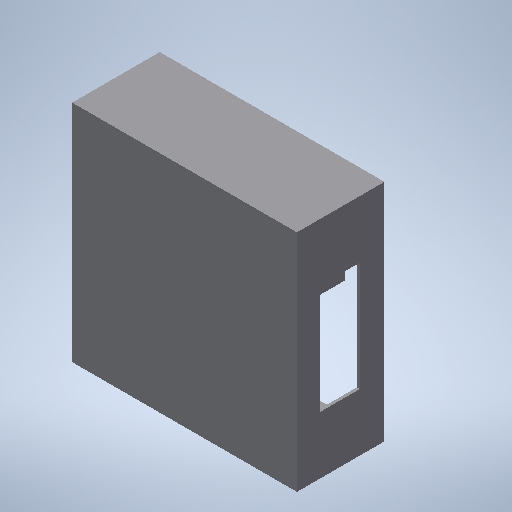
# Autodesk Inventor part: 零件1
Saved by Autodesk Inventor 2025 (Build 290162000, 162)
## iProperties
Created: 2024-03-26
Part Number: 零件1
Material: 常规
Document SubType Name: Modeling
Designer: Administrator
Density: 1 g/cm^3
Appearance: 默认
Author: Administrator
Autodesk Inventor part; units mm, degrees
ref_plane "YZ Plane" through (0, 0, 0) normal (1, 0, 0) x (0, 1, 0)
ref_plane "XZ Plane" through (0, 0, 0) normal (0, 1, 0) x (-1, 0, 0)
ref_plane "XY Plane" through (0, 0, 0) normal (0, 0, 1) x (1, 0, 0)
sketch "草图1" plane through (0, 0, 0) normal (0, 1, 0) x (-1, 0, 0)
  line L0 (75, 0) -> (75, -75)
  line L1 (75, -75) -> (-75, -75)
  line L2 (-75, -75) -> (-75, 75)
  line L3 (-75, 75) -> (75, 75)
  line L4 (75, 75) -> (75, 0)
  line L5 (77, 0) -> (77, 77)
  line L6 (77, 77) -> (-77, 77)
  line L7 (-77, 77) -> (-77, -77)
  line L8 (-77, -77) -> (77, -77)
  line L9 (77, -77) -> (77, 0)
  line L10 (75, 0) -> (75, 27)
  line L11 (75, 27) -> (7, 27)
  line L12 (7, 27) -> (7, -27)
  line L13 (7, -27) -> (75, -27)
  line L14 (75, -27) -> (75, -29)
  line L15 (75, -29) -> (5, -29)
  line L16 (5, -29) -> (5, 29)
  line L17 (5, 29) -> (75, 29)
  point P0 (0, 0)
  dimension "d2" = 150
  dimension "d3" = 150
  dimension "d4" = 150
  dimension "d6" = 77
  dimension "d7" = 154
  dimension "d8" = 154
  dimension "d9" = 154
  dimension "d14" = 70
  constraints: 36 end point, 6 perpendicular, 4 parallel, 4 point on line
  measures "d2" distance of L0.end L1.end
  measures "d3" distance of L1.end L2.end
  measures "d4" distance of L2.end L3.end
  measures "d6" distance of L5.start L5.end
  measures "d7" distance of L5.end L6.end
  measures "d8" distance of L6.end L7.end
  measures "d9" distance of L7.end L8.end
  measures "d14" distance of L14.end L15.end
sketch "草图2" plane through (0, 0, 0) normal (0, 1, 0) x (-1, 0, 0)
  line L0 (75, 0) -> (75, -75)
  line L1 (75, -75) -> (-75, -75)
  line L2 (-75, -75) -> (-75, 75)
  line L3 (-75, 75) -> (75, 75)
  line L4 (75, 75) -> (75, 0)
  line L5 (77, 0) -> (77, 77)
  line L6 (77, 77) -> (-77, 77)
  line L7 (-77, 77) -> (-77, -77)
  line L8 (-77, -77) -> (77, -77)
  line L9 (77, -77) -> (77, 0)
  line L10 (75, 0) -> (75, 27)
  line L11 (75, 27) -> (7, 27)
  line L12 (7, 27) -> (7, -27)
  line L13 (7, -27) -> (75, -27)
  line L14 (75, -27) -> (75, -29)
  line L15 (75, -29) -> (5, -29)
  line L16 (5, -29) -> (5, 29)
  line L17 (5, 29) -> (75, 29)
  line L18 (75, 0) -> (75, -75)
  line L19 (75, -75) -> (-75, -75)
  line L20 (-75, -75) -> (-75, 75)
  line L21 (-75, 75) -> (75, 75)
  line L22 (75, 75) -> (75, 0)
  line L23 (77, 0) -> (77, 77)
  line L24 (77, 77) -> (-77, 77)
  line L25 (-77, 77) -> (-77, -77)
  line L26 (-77, -77) -> (77, -77)
  line L27 (77, -77) -> (77, 0)
  line L28 (75, 0) -> (75, 27)
  line L29 (75, 27) -> (7, 27)
  line L30 (7, 27) -> (7, -27)
  line L31 (7, -27) -> (75, -27)
  line L32 (75, -27) -> (75, -29)
  line L33 (75, -29) -> (5, -29)
  line L34 (5, -29) -> (5, 29)
  line L35 (5, 29) -> (75, 29)
  point P0 (0, 0)
  point P1 (0, 0)
  point P2 (0, 0)
  dimension "d16" = 150
  dimension "d17" = 150
  dimension "d18" = 150
  dimension "d19" = 77
  dimension "d20" = 154
  dimension "d21" = 154
  dimension "d22" = 154
  dimension "d23" = 70
  dimension "d24" = 150
  dimension "d25" = 150
  dimension "d26" = 150
  dimension "d27" = 77
  dimension "d28" = 154
  dimension "d29" = 154
  dimension "d30" = 154
  dimension "d31" = 70
  constraints: 72 end point, 12 perpendicular, 8 parallel, 8 point on line
  measures "d16" distance of L0.end L1.end
  measures "d17" distance of L1.end L2.end
  measures "d18" distance of L2.end L3.end
  measures "d19" distance of L5.start L5.end
  measures "d20" distance of L5.end L6.end
  measures "d21" distance of L6.end L7.end
  measures "d22" distance of L7.end L8.end
  measures "d23" distance of L14.end L15.end
  measures "d24" distance of L18.end L19.end
  measures "d25" distance of L19.end L20.end
  measures "d26" distance of L20.end L21.end
  measures "d27" distance of L23.start L23.end
  measures "d28" distance of L23.end L24.end
  measures "d29" distance of L24.end L25.end
  measures "d30" distance of L25.end L26.end
  measures "d31" distance of L32.end L33.end
sketch "草图3" plane through (0, 0, 0) normal (0, 1, 0) x (-1, 0, 0)
  line L0 (75, 0) -> (75, -75)
  line L1 (75, -75) -> (-75, -75)
  line L2 (-75, -75) -> (-75, 75)
  line L3 (-75, 75) -> (75, 75)
  line L4 (75, 75) -> (75, 0)
  line L5 (77, 0) -> (77, 77)
  line L6 (77, 77) -> (-77, 77)
  line L7 (-77, 77) -> (-77, -77)
  line L8 (-77, -77) -> (77, -77)
  line L9 (77, -77) -> (77, 0)
  line L10 (75, 0) -> (75, 27)
  line L11 (75, 27) -> (7, 27)
  line L12 (7, 27) -> (7, -27)
  line L13 (7, -27) -> (75, -27)
  line L14 (75, -27) -> (75, -29)
  line L15 (75, -29) -> (5, -29)
  line L16 (5, -29) -> (5, 29)
  line L17 (5, 29) -> (75, 29)
  point P0 (0, 0)
  point P1 (0, 0)
  dimension "d32" = 150
  dimension "d33" = 150
  dimension "d34" = 150
  dimension "d35" = 77
  dimension "d36" = 154
  dimension "d37" = 154
  dimension "d38" = 154
  dimension "d39" = 70
  constraints: 36 end point, 6 perpendicular, 4 parallel, 4 point on line
  measures "d32" distance of L0.end L1.end
  measures "d33" distance of L1.end L2.end
  measures "d34" distance of L2.end L3.end
  measures "d35" distance of L5.start L5.end
  measures "d36" distance of L5.end L6.end
  measures "d37" distance of L6.end L7.end
  measures "d38" distance of L7.end L8.end
  measures "d39" distance of L14.end L15.end
extrude "拉伸3" add sketch "草图3" along normal blind 5 contours L0 L15 L16 L17 L4 L11 L12 L13 | L9 L8 L7 L6 L5
extrude "拉伸4" add sketch "草图2" along normal blind 50
extrude "拉伸5" add sketch "草图1" against normal blind 10 contours L0 L13 L12 L11 L4 | L0 L15 L16 L17 L4 L11 L12 L13 | L0 L1 L2 L3 L4 L17 L16 L15 | L9 L8 L7 L6 L5
sketch "草图4" plane through (77, 50, 77) normal (1, 0, 0) x (0, 0, -1)
  line L0 (77, -44) -> (114.5, -44)
  line L1 (114.5, -44) -> (114.5, -17)
  line L2 (114.5, -17) -> (39.5, -17)
  line L3 (39.5, -17) -> (39.5, -44)
  line L4 (39.5, -44) -> (77, -44)
  point P0 (77, -50)
  dimension "d53" = 27
  dimension "d54" = 75
  constraints: 10 end point
  measures "d53" distance of L0.end L1.end
  measures "d54" distance of L1.end L2.end
extrude "拉伸6" cut sketch "草图4" against normal blind 3
sketch "草图5" plane through (-77, 50, -77) normal (-1, 0, 0) x (0, 0, 1)
  line L0 (154, -60) -> (0, -60) projected
  line L1 (77, -50) -> (104, -50)
  line L2 (104, -50) -> (104, -40)
  line L3 (104, -40) -> (50, -40)
  line L4 (50, -40) -> (50, -50)
  line L5 (50, -50) -> (77, -50)
  dimension "d58" = 10
  dimension "d59" = 54
  constraints: 10 end point, 2 parallel, 2 perpendicular, 1 collinear
  measures "d58" distance of L1.end L2.end
  measures "d59" distance of L2.end L3.end
extrude "拉伸7" cut sketch "草图5" against normal blind 2
sketch "草图6" plane through (0, 0, 0) normal (0, 1, 0) x (1, 0, 0)
  line L0 (75, -75) -> (75, 75) projected
  line L1 (0, 0) -> (0, 15)
  line L2 (0, 15) -> (30, 15)
  line L3 (30, 15) -> (30, -15)
  line L4 (30, -15) -> (0, -15)
  line L5 (0, -15) -> (0, 0)
  line L6 (0, -15) -> (0, -9)
  line L7 (0, -15) -> (7, -15)
  line L8 (7, -15) -> (7, -9)
  line L9 (7, -9) -> (10, -9)
  line L10 (10, -9) -> (10, -15)
  constraints: 20 end point, 4 parallel, 3 perpendicular, 3 point on line, 1 collinear
sketch "草图7" plane through (0, 0, 0) normal (0, 1, 0) x (1, 0, 0)
  line L0 (75, 75) -> (-75, 75)
  line L1 (-75, 75) -> (-75, 29)
  line L2 (-75, 29) -> (-5, 29)
  line L3 (-5, 29) -> (-5, -29)
  line L4 (-5, -29) -> (-75, -29)
  line L5 (-75, -29) -> (-75, -75)
  line L6 (-75, -75) -> (75, -75)
  line L7 (75, -75) -> (75, 75)
  line L8 (0, 0) -> (0, 15)
  line L9 (0, 15) -> (30, 15)
  line L10 (30, 15) -> (30, -15)
  line L11 (30, -15) -> (0, -15)
  line L12 (0, -15) -> (0, 0)
  line L13 (0, -15) -> (0, -9)
  line L14 (0, -15) -> (7, -15)
  line L15 (7, -15) -> (7, -9)
  line L16 (7, -9) -> (10, -9)
  line L17 (10, -9) -> (10, -15)
  constraints: 36 end point, 4 parallel, 3 perpendicular, 3 point on line, 1 collinear
extrude "拉伸8" add sketch "草图7" along normal blind 70 contours L8 L9 L10 L11 L17 L16 L15 L12 | L15 L16 L17 L11
extrude "拉伸9" add sketch "草图6" along normal blind 87.9 contours L8 L9 L10 L4
sketch "草图8" plane through (10, 70, 9) normal (1, 0, 0) x (0, 0, -1)
  line L0 (0, 0) -> (0, 17.9) projected
  line L1 (0, 0) -> (0, 5)
  circle A0 centre (-3, 12.9) radius 1.5
  circle A1 centre (-3, 5) radius 1.5
  dimension "d80" = 3
  dimension "d81" = 3
  constraints: 2 centre point, 2 end point, 1 point on line
  measures "d80" diameter of A0
  measures "d81" diameter of A1
extrude "拉伸11" cut sketch "草图8" against normal blind 10
